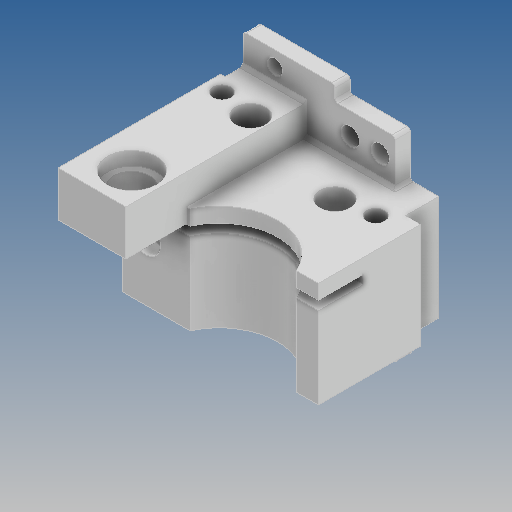
# Autodesk Inventor part: 0008-30-005
Saved by Autodesk Inventor 2020 (Build 240168000, 168)
## iProperties
Created: 2021-05-22
Part Number: 0008-30-005
Material: Generic
Document SubType Name: Modeling
Designer: Iulian Bors
Density: 1 g/cm^3
Appearance: Default
Author: Iulian Bors
Subject: 005
Autodesk Inventor part; units mm, degrees
ref_plane "YZ Plane" through (0, 0, 0) normal (1, 0, 0) x (0, 1, 0)
ref_plane "XZ Plane" through (0, 0, 0) normal (0, 1, 0) x (-1, 0, 0)
ref_plane "XY Plane" through (0, 0, 0) normal (0, 0, 1) x (1, 0, 0)
sketch "Sketch1" plane through (0, 0, 0) normal (0, 0, 1) x (1, 0, 0)
  line L0 (-32.5, 17.5) -> (32.5, 17.5)
  line L1 (32.5, 17.5) -> (32.5, -17.5)
  line L2 (32.5, -17.5) -> (-32.5, -17.5)
  line L3 (-32.5, -17.5) -> (-32.5, 17.5)
  point P0 (0, 0)
  point P1 (0, 17.5)
  point P2 (-32.5, 0)
  dimension "d0" = 65
  dimension "d1" = 35
  constraints: 8 end point, 2 midpoint, 2 parallel, 1 horizontal, 1 horizontal alignment, 1 perpendicular, 1 vertical alignment
  measures "d0" distance of L0.start L0.end
  measures "d1" distance of L2.end L0.start
extrude "Extrusion1" add sketch "Sketch1" along normal blind 45
sketch "Sketch3" plane through (0, 0, 45) normal (0, 0, 1) x (1, 0, 0)
  line L0 (-32.5, 12.5) -> (32.5, 12.5)
  line L1 (32.5, 12.5) -> (32.5, 9.6)
  line L2 (32.5, 9.6) -> (-32.5, 9.6)
  line L3 (-32.5, 9.6) -> (-32.5, 12.5)
  line L4 (32.5, -17.5) -> (32.5, 17.5) projected
  line L5 (-32.5, 17.5) -> (-32.5, -17.5) projected
  line L6 (32.5, 17.5) -> (-32.5, 17.5) projected
  point P0 (0, 0)
  point P1 (45, 15)
  point P2 (-45, 15)
  dimension "d8" = 2.9
  dimension "d9" = 5
  constraints: 8 end point, 2 parallel, 2 vertical, 1 horizontal, 1 perpendicular, 2 other
  measures "d8" distance between parallel lines of L2 L0
  measures "d9" distance between parallel lines of L0 L6
extrude "Extrusion3" cut sketch "Sketch3" against normal blind 15 contours L0 L1 L2 L3
sketch "Sketch4" plane through (-11.5, -17.5, 0) normal (0, -1, 0) x (1, 0, 0)
  circle A0 centre (19, 53) radius 19.4
  line L0 (-21, 45) -> (44, 45) projected
  line L1 (44, 0) -> (44, 45) projected
  point P0 (24, 0)
  point P1 (19, 0)
  dimension "d12" = 38.8
  dimension "d16" = 8
  dimension "d17" = 25
  constraints: 1 centre point, 1 vertical alignment
  measures "d12" diameter of A0
  measures "d16" distance from line of L0 A0.centre
  measures "d17" distance from line of L1 A0.centre
extrude "Extrusion4" cut sketch "Sketch4" against normal through all
sketch "Sketch6" plane through (-32.5, -17.5, 0) normal (0, -1, 0) x (1, 0, 0)
  line L0 (60, 11) -> (65, 11)
  line L1 (65, 11) -> (65, 0)
  line L2 (65, 0) -> (60, 0)
  line L3 (60, 0) -> (60, 11)
  line L4 (0, 0) -> (65, 0) projected
  line L5 (65, 0) -> (65, 45) projected
  point P0 (32.5, 0)
  dimension "d18" = 5
  dimension "d19" = 11
  constraints: 8 end point, 2 collinear, 2 parallel, 1 horizontal, 1 perpendicular
  measures "d18" distance of L0.start L0.end
  measures "d19" distance of L2.end L0.start
extrude "Extrusion5" cut sketch "Sketch6" against normal through all
sketch "Sketch7" plane through (-32.5, 17.5, 45) normal (0, 1, 0) x (1, 0, 0)
  line L0 (0, 45) -> (21, 45)
  line L1 (21, 45) -> (21, -20)
  line L2 (21, -20) -> (0, -20)
  line L3 (0, -20) -> (0, 45)
  line L4 (0, 45) -> (0, 0) projected
  line L5 (22.3263, 0) -> (0, 0) projected
  line L6 (60, 45) -> (0, 45) projected
  point P0 (32.5, 45)
  dimension "d22" = 21
  dimension "d24" = 20
  constraints: 8 end point, 2 collinear, 2 parallel, 1 horizontal, 1 perpendicular
  measures "d22" distance of L0.start L0.end
  measures "d24" distance between parallel lines of L2 L5
extrude "Extrusion6" add sketch "Sketch7" along normal blind 10
move faces "Move1" translate (0, -5, 0) faces at (-18.5, 17.5, 58.3333)
sketch "Sketch9" plane through (-32.5, 27.5, 45) normal (0, 1, 0) x (1, 0, 0)
  circle A0 centre (11.5, -8.5) radius 8 projected
  point P0 (32.5, 45)
hole "Hole1" at (-21, 27.5, 53.5) direction (0, -1, 0) diameter 12 end through all counterbore diameter 16.3 counterbore depth 4.5
sketch "Sketch10" plane through (-32.5, -17.5, 0) normal (0, -1, 0) x (1, 0, 0)
  line L0 (0, 0) -> (60, 0) projected
  circle A0 centre (15.5, 18) radius 4 projected
  arc A1 (42.5, 22.0277) -> (44.5, 22.0277) centre (43.5, 18) ccw projected
  point P0 (32.5, 0)
hole "Hole2" at (-17, -17.5, 18) at (11, -17.5, 18) direction (0, 1, 0) diameter 10 end through all
sketch "Sketch11" plane through (-32.5, -17.5, 0) normal (0, -1, 0) x (1, 0, 0)
  circle A0 centre (55.0422, 16) radius 2.5 projected
  circle A1 centre (3.9578, 16) radius 2.5 projected
  circle A2 centre (55.0422, 16) radius 2.5 projected
  circle A3 centre (3.9578, 16) radius 2.5 projected
  point P0 (32.5, 0)
hole "Hole3" at (22.5422, -17.5, 16) at (-28.5422, -17.5, 16) direction (0, 1, 0) diameter 6 end through all
sketch "Sketch13" plane through (-32.5, -17.5, 0) normal (0, -1, 0) x (1, 0, 0)
  line L0 (0, 35) -> (15, 35)
  line L1 (15, 35) -> (15, 25)
  line L2 (15, 25) -> (0, 25)
  line L3 (0, 25) -> (0, 35)
  line L4 (0, 0) -> (0, 45) projected
  line L5 (0, 45) -> (22.3263, 45) projected
  point P0 (32.5, 0)
  dimension "d53" = 10
  dimension "d54" = 15
  dimension "d55" = 10
  constraints: 8 end point, 2 parallel, 1 collinear, 1 horizontal, 1 perpendicular
  measures "d53" distance between parallel lines of L2 L0
  measures "d54" distance of L0.start L0.end
  measures "d55" distance between parallel lines of L0 L5
extrude "Extrusion7" cut sketch "Sketch13" against normal up to surface (27.1 mm away)
sketch "Sketch14" plane through (0, 0, 45) normal (0, 0, 1) x (1, 0, 0)
  line L0 (-32.5, 9.6) -> (-32.5, -17.5) projected
  line L1 (-10.1737, 9.6) -> (-32.5, 9.6) projected
  point P0 (0, 0)
  point P1 (-25, 2.05)
  dimension "d58" = 7.5
  dimension "d92" = 7.55
  measures "d58" distance from line of L0 point (-25, 2.05)
  measures "d92" distance from line of point (-25, 2.05) L1
hole "Hole4" at (-25, 2.05, 45) direction (0, 0, -1) diameter 5 depth 10 counterbore diameter 10 counterbore depth 5
sketch "Sketch15" plane through (0, 0, 0) normal (0, 0, -1) x (-1, 0, 0)
  circle A0 centre (25, 2.05) radius 2.5 projected
  point P0 (0, 0)
hole "Hole5" at (-25, 2.05, 0) direction (0, 0, 1) diameter 10 depth 25
sketch "Sketch16" plane through (0, 0, 0) normal (0, 0, -1) x (-1, 0, 0)
  line L0 (-18, 32.5) -> (2, 32.5)
  line L1 (2, 32.5) -> (2, 17.5)
  line L2 (2, 17.5) -> (-18, 17.5)
  line L3 (-18, 17.5) -> (-18, 32.5)
  line L4 (-18.5, -17.5) -> (3.5, -17.5)
  line L5 (3.5, -17.5) -> (3.5, -32.5)
  line L6 (3.5, -32.5) -> (-18.5, -32.5)
  line L7 (-18.5, -32.5) -> (-18.5, -17.5)
  line L8 (-27.5, 17.5) -> (11.5, 17.5) projected
  line L9 (10.1737, -17.5) -> (-25.1737, -17.5) projected
  line L10 (32.5, -17.5) -> (-27.5, -17.5) projected
  circle A0 centre (-13, 25) radius 3
  circle A1 centre (-3, 25) radius 3
  circle A2 centre (-12.5, -25) radius 3
  circle A3 centre (-2.5, -25) radius 3
  point P0 (0, 0)
  point P1 (-8, 32.5)
  point P2 (-8, 17.5)
  point P3 (-7.5, -32.5)
  point P4 (-7.5, -17.5)
  point P5 (2, 25)
  point P6 (3.5, -25)
  dimension "d74" = 15
  dimension "d75" = 10
  dimension "d76" = 5
  dimension "d77" = 5
  dimension "d78" = 6
  dimension "d79" = 10
  dimension "d80" = 6
  dimension "d81" = 6
  constraints: 16 end point, 6 midpoint, 5 parallel, 4 centre point, 4 horizontal alignment, 3 equal radius, 2 collinear, 2 horizontal, 2 perpendicular, 2 vertical alignment
  measures "d74" distance of L2.end L0.start
  measures "d75" distance of A1.centre A0.centre
  measures "d76" distance from line of A0.centre L3
  measures "d77" distance from line of A1.centre L1
  measures "d78" diameter of A0
  measures "d79" distance of A3.centre A2.centre
  measures "d80" distance from line of L5 A3.centre
  measures "d81" distance from line of A2.centre L7
extrude "Extrusion8" add sketch "Sketch16" against normal blind 5
sketch "Sketch18" plane through (0, 0, 0) normal (0, 0, -1) x (-1, 0, 0)
  line L0 (2, 37.5) -> (32.5, 37.5)
  line L1 (32.5, 37.5) -> (32.5, 27.5)
  line L2 (32.5, 27.5) -> (2, 27.5)
  line L3 (2, 27.5) -> (2, 37.5)
  line L4 (3.5, -17.5) -> (32.5, -17.5)
  line L5 (32.5, -17.5) -> (32.5, -27.5)
  line L6 (32.5, -27.5) -> (3.5, -27.5)
  line L7 (3.5, -27.5) -> (3.5, -17.5)
  line L8 (11.5, 27.5) -> (32.5, 27.5) projected
  line L9 (32.5, 27.5) -> (32.5, -17.5) projected
  line L10 (11.5, 17.5) -> (11.5, 27.5) projected
  line L11 (32.5, -17.5) -> (3.5, -17.5) projected
  circle A0 centre (22, 32.5) radius 2.5
  circle A1 centre (22, -22.5) radius 2.5
  line L12 (2, 32.5) -> (2, 17.5) projected
  line L13 (3.5, -17.5) -> (3.5, -32.5) projected
  line L14 (2, 17.5) -> (11.5, 17.5) projected
  point P0 (0, 0)
  point P1 (32.5, 32.5)
  point P2 (32.5, -22.5)
  point P3 (2, 27.5)
  dimension "d84" = 10
  dimension "d85" = 5
  dimension "d86" = 10
  dimension "d93" = 10.5
  constraints: 16 end point, 6 collinear, 4 parallel, 2 centre point, 2 horizontal, 2 horizontal alignment, 2 midpoint, 2 perpendicular, 1 equal radius, 1 vertical alignment
  measures "d84" distance between parallel lines of L2 L0
  measures "d85" diameter of A0
  measures "d86" distance of L4.end L5.end
  measures "d93" distance from line of L5 A1.centre
extrude "Extrusion9" add sketch "Sketch18" against normal blind 5
chamfer "Chamfer1" distance 1 angle 45 3 edges at (-22, 27.5, 5) (-7, -17.5, 5) (3.25, 17.5, 5)
sketch "Sketch19" plane through (-32.5, 12.5, 30) normal (-1, 0, 0) x (0, 0, 1)
  line L0 (-5, 15) -> (-19, 15)
  line L1 (-19, 15) -> (-19, -30)
  line L2 (-19, -30) -> (-5, -30)
  line L3 (-5, -30) -> (-5, 15)
  line L4 (-24, -30) -> (-5, -30) projected
  line L5 (-5, -30) -> (-5, -2.9) projected
  line L6 (-24, 15) -> (35, 15) projected
  line L7 (-20, -96.08) -> (-20, 148.92) projected
  line L8 (-30, 25) -> (-30, -40) projected
  line L9 (35, 15) -> (-5, 15)
  line L10 (-5, 15) -> (-5, 0)
  line L11 (-5, 0) -> (35, 0)
  line L12 (35, 0) -> (35, 15)
  line L13 (0, 0) -> (35, 0) projected
  line L14 (35, 0) -> (35, 15) projected
  point P0 (-30, -12.5)
  point P1 (35, 15)
  point P2 (-5, 15)
  dimension "d94" = 11
  constraints: 16 end point, 6 collinear, 4 parallel, 2 horizontal, 2 perpendicular, 1 point on line
  measures "d94" distance between parallel lines of L8 L1
extrude "Extrusion10" add sketch "Sketch19" along normal blind 1.5 contours L3 L2 L1 L0 | L6 L12 L11 L3
fillet "Fillet1" radius 1 10 edges at (-3.5, -27.5, 2.5) (-2, 32.5, 2.5) (-2, 37.5, 2.5) (18, 32.5, 2.5) (-32.5, 37.5, 2.5) (-32.5, -27.5, 2.5) (18.5, -32.5, 2.5) (-3.5, -32.5, 2.5) (18.5, -17.5, 3) (18, 17.5, 3)
equation "\"d79\" = d75"
equation "\"d80\" = d78"
equation "\"d81\" = d78"
equation "\"d86\" = d84"
body "Solid1"
